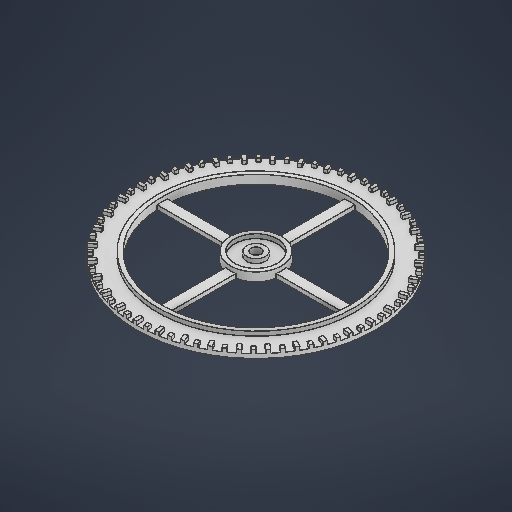
# Autodesk Inventor part: measuring_disk2
Saved by Autodesk Inventor 2026.1 (Build 301233000, 233)
## iProperties
Created: 2025-12-25
Part Number: measuring_disk2
Material: Generic
Document SubType Name: Modeling
Designer: emanuel
Density: 1 g/cm^3
Appearance: Default
Author: emanuel
Autodesk Inventor part; units mm, degrees
ref_plane "YZ Plane" through (0, 0, 0) normal (1, 0, 0) x (0, 1, 0)
ref_plane "XZ Plane" through (0, 0, 0) normal (0, 1, 0) x (-1, 0, 0)
ref_plane "XY Plane" through (0, 0, 0) normal (0, 0, 1) x (1, 0, 0)
sketch "Sketch1" plane through (0, 0, 0) normal (0, 1, 0) x (-1, 0, 0)
  circle A0 centre (0, 0) radius 3
  circle A1 centre (0, 0) radius 70
  circle A2 centre (0, 0) radius 15
  circle A3 centre (0, 0) radius 55
  line L0 (0, -3) -> (70, -3)
  line L1 (70, -3) -> (70, 3)
  line L2 (70, 3) -> (0, 3)
  line L3 (0, 3) -> (0, -3)
  line L4 (3, 0) -> (-3, 0)
  line L5 (-3, 0) -> (-3, -70)
  line L6 (-3, -70) -> (3, -70)
  line L7 (3, -70) -> (3, 0)
  line L8 (0, 3) -> (-70, 3)
  line L9 (-70, 3) -> (-70, -3)
  line L10 (-70, -3) -> (0, -3)
  line L11 (0, -3) -> (0, 3)
  line L12 (-3, 0) -> (3, 0)
  line L13 (3, 0) -> (3, 70)
  line L14 (3, 70) -> (-3, 70)
  line L15 (-3, 70) -> (-3, 0)
  point P0 (54.9181, -3)
  point P1 (3, -54.9181)
  point P2 (3, -14.6969)
  point P3 (14.6969, -3)
  point P4 (-3, -54.9181)
  point P5 (-54.9181, -3)
  point P6 (-14.6969, -3)
  point P7 (-3, -14.6969)
  point P8 (-54.9181, 3)
  point P9 (-3, 54.9181)
  point P10 (-3, 14.6969)
  point P11 (-14.6969, 3)
  point P12 (54.9181, 3)
  point P13 (14.6969, 3)
  point P14 (3, 14.6969)
  point P15 (3, 54.9181)
  dimension "d0" = 6
  dimension "d1" = 140
  dimension "d2" = 30
  dimension "d3" = 110
  dimension "d4" = 70
  dimension "d5" = 6
  dimension "d6" = 6
  dimension "d7" = 70
  dimension "d8" = 70
  dimension "d9" = 6
  dimension "d10" = 6
  dimension "d11" = 70
  constraints: 32 end point, 8 parallel, 4 centre point, 4 coincident, 4 horizontal, 4 perpendicular, 2 point on circle
  measures "d0" diameter of A0
  measures "d1" diameter of A1
  measures "d2" diameter of A2
  measures "d3" diameter of A3
  measures "d4" distance of L2.end L1.end
  measures "d5" distance of L1.end L0.end
  measures "d6" distance of L6.end L5.end
  measures "d7" distance of L5.end L4.end
  measures "d8" distance of L10.end L9.end
  measures "d9" distance of L9.end L8.end
  measures "d10" distance of L14.end L13.end
  measures "d11" distance of L13.end L12.end
extrude "Extrusion1" add sketch "Sketch1" along normal blind 2.5 contours L7 L0 A0 | L13 L2 A2 L0 L7 | A0 L2 L13 | L8 L15 A2 L13 L2 | A0 L15 L8 | L10 L5 A0 | L0 L7 A2 L5 L10 | L0 A2 L7 | L13 A2 L2 | L5 L10 A2 L8 L15 | L8 A2 L15 | L5 A2 L10 | A2 L2 A3 L0 | L7 A3 L5 A2 | A2 L15 A3 L13 | A2 L10 A3 L8 | L0 A1 L7 A3 | A3 L2 A1 L0 | L7 A1 L5 A3 | A3 L13 A1 L2 | A3 L15 A1 L13 | L8 A1 L15 A3 | A3 L10 A1 L8 | L5 A1 L10 A3
sketch "Sketch2" plane through (0, 2.5, 0) normal (0, 1, 0) x (1, 0, 0)
  circle A0 centre (0, 0) radius 3 projected
  circle A1 centre (0, 0) radius 70
  arc A2 (-3, 54.9181) -> (-54.9181, 3) centre (0, 0) ccw projected
  circle A3 centre (0, 0) radius 55
  circle A4 centre (0, 0) radius 57.5
  circle A5 centre (0, 0) radius 15
  circle A6 centre (0, 0) radius 12.5
  circle A7 centre (0, 0) radius 3
  circle A8 centre (0, 0) radius 5.5
  point P0 (14.6969, -3)
  point P1 (-3, 54.9181)
  dimension "d14" = 115
  dimension "d15" = 25
  dimension "d32" = 11
  constraints: 7 coincident, 5 centre point, 1 concentric, 6 other
  measures "d14" diameter of A4
  measures "d15" diameter of A6
  measures "d32" diameter of A8
extrude "Extrusion2" add sketch "Sketch2" along normal blind 2.5 contours A4 | A5 | A8
sketch "Sketch3" plane through (0, 2.5, 0) normal (0, 1, 0) x (1, 0, 0)
  circle A0 centre (0, 0) radius 70 projected
  line L0 (70, 0) -> (66, 0)
  line L1 (66, 0) -> (66, -2)
  line L2 (66, -2) -> (70, -2)
  line L3 (70, -2) -> (70, 0)
  circle A1 centre (0, 0) radius 3 projected
  circle A2 centre (0, 0) radius 70
  line L4 (0, 0) -> (69.7336, 6.1009)
  line L5 (0, 0) -> (70, 0) construction
  line L6 (69.7336, 6.1009) -> (67.2431, 5.883)
  line L7 (67.2431, 5.883) -> (67.4175, 3.8906)
  line L8 (67.4175, 3.8906) -> (69.9079, 4.1085)
  line L9 (65.2, 17.4703) -> (65.7176, 15.5384)
  line L10 (67.6148, 18.1173) -> (65.2, 17.4703)
  line L11 (65.7176, 15.5384) -> (68.1324, 16.1855)
  line L12 (68.9365, 12.1554) -> (64.9973, 11.4608)
  line L13 (64.9973, 11.4608) -> (65.3446, 9.4912)
  line L14 (69.2838, 10.1858) -> (68.9365, 12.1554)
  line L15 (65.3446, 9.4912) -> (69.2838, 10.1858)
  line L16 (61.1758, 28.5267) -> (62.021, 26.7141)
  line L17 (63.4415, 29.5833) -> (61.1758, 28.5267)
  line L18 (62.021, 26.7141) -> (64.2868, 27.7707)
  line L19 (65.7785, 23.9414) -> (62.0197, 22.5733)
  line L20 (62.0197, 22.5733) -> (62.7038, 20.6939)
  line L21 (66.4625, 22.062) -> (65.7785, 23.9414)
  line L22 (62.7038, 20.6939) -> (66.4625, 22.062)
  line L23 (55.2928, 38.7164) -> (56.4399, 37.0781)
  line L24 (57.3406, 40.1504) -> (55.2928, 38.7164)
  line L25 (56.4399, 37.0781) -> (58.4878, 38.512)
  line L26 (60.6218, 35) -> (57.1577, 33)
  line L27 (57.1577, 33) -> (58.1577, 31.2679)
  line L28 (61.6218, 33.2679) -> (60.6218, 35)
  line L29 (58.1577, 31.2679) -> (61.6218, 33.2679)
  line L30 (47.7297, 47.7297) -> (49.1439, 46.3155)
  line L31 (49.4975, 49.4975) -> (47.7297, 47.7297)
  line L32 (49.1439, 46.3155) -> (50.9117, 48.0833)
  line L33 (53.6231, 44.9951) -> (50.5589, 42.424)
  line L34 (50.5589, 42.424) -> (51.8445, 40.8919)
  line L35 (54.9087, 43.463) -> (53.6231, 44.9951)
  line L36 (51.8445, 40.8919) -> (54.9087, 43.463)
  line L37 (38.7164, 55.2928) -> (40.3547, 54.1456)
  line L38 (40.1504, 57.3406) -> (38.7164, 55.2928)
  line L39 (40.3547, 54.1456) -> (41.7887, 56.1935)
  line L40 (44.9951, 53.6231) -> (42.424, 50.5589)
  line L41 (42.424, 50.5589) -> (43.9561, 49.2734)
  line L42 (46.5272, 52.3375) -> (44.9951, 53.6231)
  line L43 (43.9561, 49.2734) -> (46.5272, 52.3375)
  line L44 (28.5267, 61.1758) -> (30.3393, 60.3305)
  line L45 (29.5833, 63.4415) -> (28.5267, 61.1758)
  line L46 (30.3393, 60.3305) -> (31.3959, 62.5963)
  line L47 (35, 60.6218) -> (33, 57.1577)
  line L48 (33, 57.1577) -> (34.7321, 56.1577)
  line L49 (36.7321, 59.6218) -> (35, 60.6218)
  line L50 (34.7321, 56.1577) -> (36.7321, 59.6218)
  line L51 (17.4703, 65.2) -> (19.4021, 64.6824)
  line L52 (18.1173, 67.6148) -> (17.4703, 65.2)
  line L53 (19.4021, 64.6824) -> (20.0492, 67.0972)
  line L54 (23.9414, 65.7785) -> (22.5733, 62.0197)
  line L55 (22.5733, 62.0197) -> (24.4527, 61.3357)
  line L56 (25.8208, 65.0944) -> (23.9414, 65.7785)
  line L57 (24.4527, 61.3357) -> (25.8208, 65.0944)
  line L58 (5.883, 67.2431) -> (7.8754, 67.0688)
  line L59 (6.1009, 69.7336) -> (5.883, 67.2431)
  line L60 (7.8754, 67.0688) -> (8.0933, 69.5593)
  line L61 (12.1554, 68.9365) -> (11.4608, 64.9973)
  line L62 (11.4608, 64.9973) -> (13.4304, 64.65)
  line L63 (14.125, 68.5892) -> (12.1554, 68.9365)
  line L64 (13.4304, 64.65) -> (14.125, 68.5892)
  line L65 (-5.883, 67.2431) -> (-3.8906, 67.4175)
  line L66 (-6.1009, 69.7336) -> (-5.883, 67.2431)
  line L67 (-3.8906, 67.4175) -> (-4.1085, 69.9079)
  line L68 (0, 70) -> (0, 66)
  line L69 (0, 66) -> (2, 66)
  line L70 (2, 70) -> (0, 70)
  line L71 (2, 66) -> (2, 70)
  line L72 (-17.4703, 65.2) -> (-15.5384, 65.7176)
  line L73 (-18.1173, 67.6148) -> (-17.4703, 65.2)
  line L74 (-15.5384, 65.7176) -> (-16.1855, 68.1324)
  line L75 (-12.1554, 68.9365) -> (-11.4608, 64.9973)
  line L76 (-11.4608, 64.9973) -> (-9.4912, 65.3446)
  line L77 (-10.1858, 69.2838) -> (-12.1554, 68.9365)
  line L78 (-9.4912, 65.3446) -> (-10.1858, 69.2838)
  line L79 (-28.5267, 61.1758) -> (-26.7141, 62.021)
  line L80 (-29.5833, 63.4415) -> (-28.5267, 61.1758)
  line L81 (-26.7141, 62.021) -> (-27.7707, 64.2868)
  line L82 (-23.9414, 65.7785) -> (-22.5733, 62.0197)
  line L83 (-22.5733, 62.0197) -> (-20.6939, 62.7038)
  line L84 (-22.062, 66.4625) -> (-23.9414, 65.7785)
  line L85 (-20.6939, 62.7038) -> (-22.062, 66.4625)
  line L86 (-38.7164, 55.2928) -> (-37.0781, 56.4399)
  line L87 (-40.1504, 57.3406) -> (-38.7164, 55.2928)
  line L88 (-37.0781, 56.4399) -> (-38.512, 58.4878)
  line L89 (-35, 60.6218) -> (-33, 57.1577)
  line L90 (-33, 57.1577) -> (-31.2679, 58.1577)
  line L91 (-33.2679, 61.6218) -> (-35, 60.6218)
  line L92 (-31.2679, 58.1577) -> (-33.2679, 61.6218)
  line L93 (-47.7297, 47.7297) -> (-46.3155, 49.1439)
  line L94 (-49.4975, 49.4975) -> (-47.7297, 47.7297)
  line L95 (-46.3155, 49.1439) -> (-48.0833, 50.9117)
  line L96 (-44.9951, 53.6231) -> (-42.424, 50.5589)
  line L97 (-42.424, 50.5589) -> (-40.8919, 51.8445)
  line L98 (-43.463, 54.9087) -> (-44.9951, 53.6231)
  line L99 (-40.8919, 51.8445) -> (-43.463, 54.9087)
  line L100 (-55.2928, 38.7164) -> (-54.1456, 40.3547)
  line L101 (-57.3406, 40.1504) -> (-55.2928, 38.7164)
  line L102 (-54.1456, 40.3547) -> (-56.1935, 41.7887)
  line L103 (-53.6231, 44.9951) -> (-50.5589, 42.424)
  line L104 (-50.5589, 42.424) -> (-49.2734, 43.9561)
  line L105 (-52.3375, 46.5272) -> (-53.6231, 44.9951)
  line L106 (-49.2734, 43.9561) -> (-52.3375, 46.5272)
  line L107 (-61.1758, 28.5267) -> (-60.3305, 30.3393)
  line L108 (-63.4415, 29.5833) -> (-61.1758, 28.5267)
  line L109 (-60.3305, 30.3393) -> (-62.5963, 31.3959)
  line L110 (-60.6218, 35) -> (-57.1577, 33)
  line L111 (-57.1577, 33) -> (-56.1577, 34.7321)
  line L112 (-59.6218, 36.7321) -> (-60.6218, 35)
  line L113 (-56.1577, 34.7321) -> (-59.6218, 36.7321)
  line L114 (-65.2, 17.4703) -> (-64.6824, 19.4021)
  line L115 (-67.6148, 18.1173) -> (-65.2, 17.4703)
  line L116 (-64.6824, 19.4021) -> (-67.0972, 20.0492)
  line L117 (-65.7785, 23.9414) -> (-62.0197, 22.5733)
  line L118 (-62.0197, 22.5733) -> (-61.3357, 24.4527)
  line L119 (-65.0944, 25.8208) -> (-65.7785, 23.9414)
  line L120 (-61.3357, 24.4527) -> (-65.0944, 25.8208)
  line L121 (-67.2431, 5.883) -> (-67.0688, 7.8754)
  line L122 (-69.7336, 6.1009) -> (-67.2431, 5.883)
  line L123 (-67.0688, 7.8754) -> (-69.5593, 8.0933)
  line L124 (-68.9365, 12.1554) -> (-64.9973, 11.4608)
  line L125 (-64.9973, 11.4608) -> (-64.65, 13.4304)
  line L126 (-68.5892, 14.125) -> (-68.9365, 12.1554)
  line L127 (-64.65, 13.4304) -> (-68.5892, 14.125)
  line L128 (-67.2431, -5.883) -> (-67.4175, -3.8906)
  line L129 (-69.7336, -6.1009) -> (-67.2431, -5.883)
  line L130 (-67.4175, -3.8906) -> (-69.9079, -4.1085)
  line L131 (-70, 0) -> (-66, 0)
  line L132 (-66, 0) -> (-66, 2)
  line L133 (-70, 2) -> (-70, 0)
  line L134 (-66, 2) -> (-70, 2)
  line L135 (-65.2, -17.4703) -> (-65.7176, -15.5384)
  line L136 (-67.6148, -18.1173) -> (-65.2, -17.4703)
  line L137 (-65.7176, -15.5384) -> (-68.1324, -16.1855)
  line L138 (-68.9365, -12.1554) -> (-64.9973, -11.4608)
  line L139 (-64.9973, -11.4608) -> (-65.3446, -9.4912)
  line L140 (-69.2838, -10.1858) -> (-68.9365, -12.1554)
  line L141 (-65.3446, -9.4912) -> (-69.2838, -10.1858)
  line L142 (-61.1758, -28.5267) -> (-62.021, -26.7141)
  line L143 (-63.4415, -29.5833) -> (-61.1758, -28.5267)
  line L144 (-62.021, -26.7141) -> (-64.2868, -27.7707)
  line L145 (-65.7785, -23.9414) -> (-62.0197, -22.5733)
  line L146 (-62.0197, -22.5733) -> (-62.7038, -20.6939)
  line L147 (-66.4625, -22.062) -> (-65.7785, -23.9414)
  line L148 (-62.7038, -20.6939) -> (-66.4625, -22.062)
  line L149 (-55.2928, -38.7164) -> (-56.4399, -37.0781)
  line L150 (-57.3406, -40.1504) -> (-55.2928, -38.7164)
  line L151 (-56.4399, -37.0781) -> (-58.4878, -38.512)
  line L152 (-60.6218, -35) -> (-57.1577, -33)
  line L153 (-57.1577, -33) -> (-58.1577, -31.2679)
  line L154 (-61.6218, -33.2679) -> (-60.6218, -35)
  line L155 (-58.1577, -31.2679) -> (-61.6218, -33.2679)
  line L156 (-47.7297, -47.7297) -> (-49.1439, -46.3155)
  line L157 (-49.4975, -49.4975) -> (-47.7297, -47.7297)
  line L158 (-49.1439, -46.3155) -> (-50.9117, -48.0833)
  line L159 (-53.6231, -44.9951) -> (-50.5589, -42.424)
  line L160 (-50.5589, -42.424) -> (-51.8445, -40.8919)
  line L161 (-54.9087, -43.463) -> (-53.6231, -44.9951)
  line L162 (-51.8445, -40.8919) -> (-54.9087, -43.463)
  line L163 (-38.7164, -55.2928) -> (-40.3547, -54.1456)
  line L164 (-40.1504, -57.3406) -> (-38.7164, -55.2928)
  line L165 (-40.3547, -54.1456) -> (-41.7887, -56.1935)
  line L166 (-44.9951, -53.6231) -> (-42.424, -50.5589)
  line L167 (-42.424, -50.5589) -> (-43.9561, -49.2734)
  line L168 (-46.5272, -52.3375) -> (-44.9951, -53.6231)
  line L169 (-43.9561, -49.2734) -> (-46.5272, -52.3375)
  line L170 (-28.5267, -61.1758) -> (-30.3393, -60.3305)
  line L171 (-29.5833, -63.4415) -> (-28.5267, -61.1758)
  line L172 (-30.3393, -60.3305) -> (-31.3959, -62.5963)
  line L173 (-35, -60.6218) -> (-33, -57.1577)
  line L174 (-33, -57.1577) -> (-34.7321, -56.1577)
  line L175 (-36.7321, -59.6218) -> (-35, -60.6218)
  line L176 (-34.7321, -56.1577) -> (-36.7321, -59.6218)
  line L177 (-17.4703, -65.2) -> (-19.4021, -64.6824)
  line L178 (-18.1173, -67.6148) -> (-17.4703, -65.2)
  line L179 (-19.4021, -64.6824) -> (-20.0492, -67.0972)
  line L180 (-23.9414, -65.7785) -> (-22.5733, -62.0197)
  line L181 (-22.5733, -62.0197) -> (-24.4527, -61.3357)
  line L182 (-25.8208, -65.0944) -> (-23.9414, -65.7785)
  line L183 (-24.4527, -61.3357) -> (-25.8208, -65.0944)
  line L184 (-5.883, -67.2431) -> (-7.8754, -67.0688)
  line L185 (-6.1009, -69.7336) -> (-5.883, -67.2431)
  line L186 (-7.8754, -67.0688) -> (-8.0933, -69.5593)
  line L187 (-12.1554, -68.9365) -> (-11.4608, -64.9973)
  line L188 (-11.4608, -64.9973) -> (-13.4304, -64.65)
  line L189 (-14.125, -68.5892) -> (-12.1554, -68.9365)
  line L190 (-13.4304, -64.65) -> (-14.125, -68.5892)
  line L191 (5.883, -67.2431) -> (3.8906, -67.4175)
  line L192 (6.1009, -69.7336) -> (5.883, -67.2431)
  line L193 (3.8906, -67.4175) -> (4.1085, -69.9079)
  line L194 (0, -70) -> (0, -66)
  line L195 (0, -66) -> (-2, -66)
  line L196 (-2, -70) -> (0, -70)
  line L197 (-2, -66) -> (-2, -70)
  line L198 (17.4703, -65.2) -> (15.5384, -65.7176)
  line L199 (18.1173, -67.6148) -> (17.4703, -65.2)
  line L200 (15.5384, -65.7176) -> (16.1855, -68.1324)
  line L201 (12.1554, -68.9365) -> (11.4608, -64.9973)
  line L202 (11.4608, -64.9973) -> (9.4912, -65.3446)
  line L203 (10.1858, -69.2838) -> (12.1554, -68.9365)
  line L204 (9.4912, -65.3446) -> (10.1858, -69.2838)
  line L205 (28.5267, -61.1758) -> (26.7141, -62.021)
  line L206 (29.5833, -63.4415) -> (28.5267, -61.1758)
  line L207 (26.7141, -62.021) -> (27.7707, -64.2868)
  line L208 (23.9414, -65.7785) -> (22.5733, -62.0197)
  line L209 (22.5733, -62.0197) -> (20.6939, -62.7038)
  line L210 (22.062, -66.4625) -> (23.9414, -65.7785)
  line L211 (20.6939, -62.7038) -> (22.062, -66.4625)
  line L212 (38.7164, -55.2928) -> (37.0781, -56.4399)
  line L213 (40.1504, -57.3406) -> (38.7164, -55.2928)
  line L214 (37.0781, -56.4399) -> (38.512, -58.4878)
  line L215 (35, -60.6218) -> (33, -57.1577)
  line L216 (33, -57.1577) -> (31.2679, -58.1577)
  line L217 (33.2679, -61.6218) -> (35, -60.6218)
  line L218 (31.2679, -58.1577) -> (33.2679, -61.6218)
  line L219 (47.7297, -47.7297) -> (46.3155, -49.1439)
  line L220 (49.4975, -49.4975) -> (47.7297, -47.7297)
  line L221 (46.3155, -49.1439) -> (48.0833, -50.9117)
  line L222 (44.9951, -53.6231) -> (42.424, -50.5589)
  line L223 (42.424, -50.5589) -> (40.8919, -51.8445)
  line L224 (43.463, -54.9087) -> (44.9951, -53.6231)
  line L225 (40.8919, -51.8445) -> (43.463, -54.9087)
  line L226 (55.2928, -38.7164) -> (54.1456, -40.3547)
  line L227 (57.3406, -40.1504) -> (55.2928, -38.7164)
  line L228 (54.1456, -40.3547) -> (56.1935, -41.7887)
  line L229 (53.6231, -44.9951) -> (50.5589, -42.424)
  line L230 (50.5589, -42.424) -> (49.2734, -43.9561)
  line L231 (52.3375, -46.5272) -> (53.6231, -44.9951)
  line L232 (49.2734, -43.9561) -> (52.3375, -46.5272)
  line L233 (61.1758, -28.5267) -> (60.3305, -30.3393)
  line L234 (63.4415, -29.5833) -> (61.1758, -28.5267)
  line L235 (60.3305, -30.3393) -> (62.5963, -31.3959)
  line L236 (60.6218, -35) -> (57.1577, -33)
  line L237 (57.1577, -33) -> (56.1577, -34.7321)
  line L238 (59.6218, -36.7321) -> (60.6218, -35)
  line L239 (56.1577, -34.7321) -> (59.6218, -36.7321)
  line L240 (65.2, -17.4703) -> (64.6824, -19.4021)
  line L241 (67.6148, -18.1173) -> (65.2, -17.4703)
  line L242 (64.6824, -19.4021) -> (67.0972, -20.0492)
  line L243 (65.7785, -23.9414) -> (62.0197, -22.5733)
  line L244 (62.0197, -22.5733) -> (61.3357, -24.4527)
  line L245 (65.0944, -25.8208) -> (65.7785, -23.9414)
  line L246 (61.3357, -24.4527) -> (65.0944, -25.8208)
  line L247 (67.2431, -5.883) -> (67.0688, -7.8754)
  line L248 (69.7336, -6.1009) -> (67.2431, -5.883)
  line L249 (67.0688, -7.8754) -> (69.5593, -8.0933)
  line L250 (68.9365, -12.1554) -> (64.9973, -11.4608)
  line L251 (64.9973, -11.4608) -> (64.65, -13.4304)
  line L252 (68.5892, -14.125) -> (68.9365, -12.1554)
  line L253 (64.65, -13.4304) -> (68.5892, -14.125)
  point P0 (68.9365, 12.1554)
  point P1 (60.6218, 35)
  point P2 (53.6231, 44.9951)
  point P3 (44.9951, 53.6231)
  point P4 (35, 60.6218)
  point P5 (23.9414, 65.7785)
  point P6 (0, 70)
  point P7 (-12.1554, 68.9365)
  point P8 (-35, 60.6218)
  point P9 (-44.9951, 53.6231)
  point P10 (-53.6231, 44.9951)
  point P11 (-60.6218, 35)
  point P12 (-65.7785, 23.9414)
  point P13 (-70, 0)
  point P14 (-68.9365, -12.1554)
  point P15 (-65.7785, -23.9414)
  point P16 (-60.6218, -35)
  point P17 (-53.6231, -44.9951)
  point P18 (-44.9951, -53.6231)
  point P19 (-35, -60.6218)
  point P20 (-23.9414, -65.7785)
  point P21 (-12.1554, -68.9365)
  point P22 (0, -70)
  point P23 (12.1554, -68.9365)
  point P24 (23.9414, -65.7785)
  point P25 (35, -60.6218)
  point P26 (44.9951, -53.6231)
  point P27 (53.6231, -44.9951)
  point P28 (60.6218, -35)
  point P29 (65.7785, -23.9414)
  point P30 (68.9365, -12.1554)
  point P31 (69.8795, 4.106)
  point P32 (69.9714, -2)
  point P33 (68.1048, 16.1781)
  point P34 (69.2557, 10.1808)
  point P35 (64.2609, 27.7586)
  point P36 (66.4357, 22.0523)
  point P37 (58.4644, 38.4957)
  point P38 (61.597, 33.2537)
  point P39 (50.8915, 48.0631)
  point P40 (54.8868, 43.4447)
  point P41 (41.7723, 56.1701)
  point P42 (46.5089, 52.3156)
  point P43 (31.3838, 62.5704)
  point P44 (36.7178, 59.597)
  point P45 (20.0418, 67.0696)
  point P46 (25.811, 65.0676)
  point P47 (8.0908, 69.5308)
  point P48 (14.12, 68.5611)
  point P49 (-4.106, 69.8795)
  point P50 (2, 69.9714)
  point P51 (-16.1781, 68.1048)
  point P52 (-10.1808, 69.2557)
  point P53 (-27.7586, 64.2609)
  point P54 (-22.0523, 66.4357)
  point P55 (-38.4957, 58.4644)
  point P56 (-33.2537, 61.597)
  point P57 (-48.0631, 50.8915)
  point P58 (-43.4447, 54.8868)
  point P59 (-56.1701, 41.7723)
  point P60 (-52.3156, 46.5089)
  point P61 (-62.5704, 31.3838)
  point P62 (-59.597, 36.7178)
  point P63 (-67.0696, 20.0418)
  point P64 (-65.0676, 25.811)
  point P65 (-69.5308, 8.0908)
  point P66 (-68.5611, 14.12)
  point P67 (-69.8795, -4.106)
  point P68 (-69.9714, 2)
  point P69 (-68.1048, -16.1781)
  point P70 (-69.2557, -10.1808)
  point P71 (-64.2609, -27.7586)
  point P72 (-66.4357, -22.0523)
  point P73 (-58.4644, -38.4957)
  point P74 (-61.597, -33.2537)
  point P75 (-50.8915, -48.0631)
  point P76 (-54.8868, -43.4447)
  point P77 (-41.7723, -56.1701)
  point P78 (-46.5089, -52.3156)
  point P79 (-31.3838, -62.5704)
  point P80 (-36.7178, -59.597)
  point P81 (-20.0418, -67.0696)
  point P82 (-25.811, -65.0676)
  point P83 (-8.0908, -69.5308)
  point P84 (-14.12, -68.5611)
  point P85 (4.106, -69.8795)
  point P86 (-2, -69.9714)
  point P87 (16.1781, -68.1048)
  point P88 (10.1808, -69.2557)
  point P89 (27.7586, -64.2609)
  point P90 (22.0523, -66.4357)
  point P91 (38.4957, -58.4644)
  point P92 (33.2537, -61.597)
  point P93 (48.0631, -50.8915)
  point P94 (43.4447, -54.8868)
  point P95 (56.1701, -41.7723)
  point P96 (52.3156, -46.5089)
  point P97 (62.5704, -31.3838)
  point P98 (59.597, -36.7178)
  point P99 (67.0696, -20.0418)
  point P100 (65.0676, -25.811)
  point P101 (69.5308, -8.0908)
  point P102 (68.5611, -14.12)
  dimension "d18" = 4
  dimension "d19" = 2
  dimension "d20" = 4
  dimension "d21" = 70
  dimension "d22" = 5
  dimension "d23" = 2.5
  dimension "d24" = 2
  dimension "d25" = 2.5
  dimension "d28" = 360
  constraints: 508 end point, 4 perpendicular, 2 horizontal, 1 centre point, 1 coincident, 1 equal length, 1 point on line, 579 other
  measures "d18" distance of L0.start L0.end
  measures "d19" distance of L0.end L1.end
  measures "d20" distance of L1.end L2.end
  measures "d21" distance of L4.start L4.end
  measures "d22" angle of L5 L4
  measures "d23" distance of L4.end L6.end
  measures "d24" distance of L6.end L7.end
  measures "d25" distance of L7.end L8.end
extrude "Extrusion3" add sketch "Sketch3" along normal blind 2 contours A0 L2 L1 L0 | L8 L7 L4 A0 | A0 L249 L247 L248 | L15 L13 L12 A0 | A0 L253 L251 L250 | L11 L9 L10 A0 | A0 L242 L240 L241 | L22 L20 L19 A0 | A0 L246 L244 L243 | L18 L16 L17 A0 | A0 L235 L233 L234 | L29 L27 L26 A0 | A0 L239 L237 L236 | L25 L23 L24 A0 | A0 L228 L226 L227 | L36 L34 L33 A0 | A0 L232 L230 L229 | L32 L30 L31 A0 | A0 L221 L219 L220 | L43 L41 L40 A0 | A0 L225 L223 L222 | L39 L37 L38 A0 | A0 L214 L212 L213 | L50 L48 L47 A0 | A0 L218 L216 L215 | L46 L44 L45 A0 | A0 L207 L205 L206 | L57 L55 L54 A0 | A0 L211 L209 L208 | L53 L51 L52 A0 | A0 L200 L198 L199 | L64 L62 L61 A0 | A0 L204 L202 L201 | L60 L58 L59 A0 | A0 L193 L191 L192 | L71 L69 L68 A0 | A0 L197 L195 L194 | L67 L65 L66 A0 | A0 L186 L184 L185 | L78 L76 L75 A0 | A0 L190 L188 L187 | L74 L72 L73 A0 | A0 L179 L177 L178 | L85 L83 L82 A0 | A0 L183 L181 L180 | L81 L79 L80 A0 | A0 L172 L170 L171 | L92 L90 L89 A0 | A0 L176 L174 L173 | L88 L86 L87 A0 | A0 L165 L163 L164 | L99 L97 L96 A0 | A0 L169 L167 L166 | L95 L93 L94 A0 | A0 L158 L156 L157 | L106 L104 L103 A0 | A0 L162 L160 L159 | L102 L100 L101 A0 | A0 L151 L149 L150 | L113 L111 L110 A0 | A0 L155 L153 L152 | L109 L107 L108 A0 | A0 L144 L142 L143 | L120 L118 L117 A0 | A0 L148 L146 L145 | L116 L114 L115 A0 | A0 L137 L135 L136 | L127 L125 L124 A0 | A0 L141 L139 L138 | L123 L121 L122 A0 | A0 L130 L128 L129 | L134 L132 L131 A0
body "Solid1"
